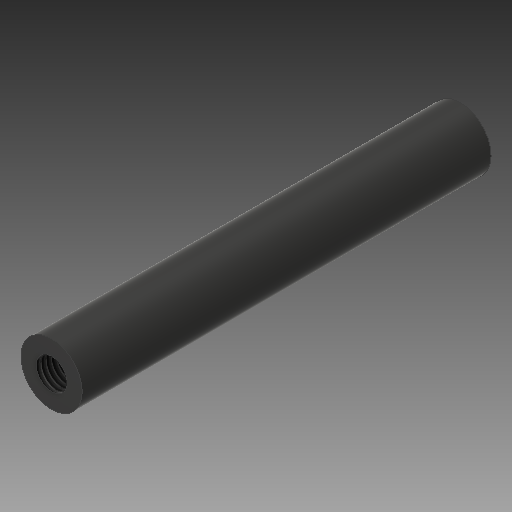
# Autodesk Inventor part: スペーサ
Saved by Autodesk Inventor 2017 (Build 210142000, 142)
## iProperties
Part Number: スペーサ
Material: 一般
Document SubType Name: Modeling
Designer: HISAAKI
Density: 1 g/cm^3
Appearance: 既定
Mass: 0.84823 g
Surface Area: 11.7338 cm^2
Volume: 0.84823 cm^3
Author: HISAAKI
Autodesk Inventor part; units mm, degrees
ref_plane "YZ Plane" through (0, 0, 0) normal (1, 0, 0) x (0, 1, 0)
ref_plane "XZ Plane" through (0, 0, 0) normal (0, 1, 0) x (-1, 0, 0)
ref_plane "XY Plane" through (0, 0, 0) normal (0, 0, 1) x (1, 0, 0)
sketch "スケッチ1" plane through (0, 0, 0) normal (0, 0, 1) x (1, 0, 0)
  circle A0 centre (0, 0) radius 3
  dimension "d0" = 6
  constraints: 1 centre point, 1 coincident
  measures "d0" diameter of A0
extrude "押し出し1" add sketch "スケッチ1" along normal blind 40
hole "穴1" at (0, 0, 40) direction (0, 0, -1) diameter 3 end through all
thread "ねじ1" size "M3x0.5" class "6H" standard "ANSI Metric M Profile" full length
